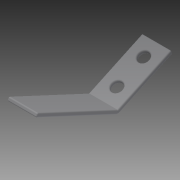
# Autodesk Inventor part: small rail
Saved by Autodesk Inventor 2014 SP1 (Build 180222100, 222)
## iProperties
Created: 2013-11-15
Part Number: small rail
Material: Polycarbonate, Clear
Document SubType Name: Modeling
Designer: RyanHughes
Density: 1.2 g/cm^3
Appearance: Polycarbonate - Clear
Author: RyanHughes
Autodesk Inventor part; units mm, degrees
ref_plane "YZ Plane" through (0, 0, 0) normal (1, 0, 0) x (0, 1, 0)
ref_plane "XZ Plane" through (0, 0, 0) normal (0, 1, 0) x (-1, 0, 0)
ref_plane "XY Plane" through (0, 0, 0) normal (0, 0, 1) x (1, 0, 0)
sketch "Sketch1" plane through (0, 0, 0) normal (0, 1, 0) x (-1, 0, 0)
  line L0 (6.35, -31.75) -> (-6.35, -31.75)
  line L1 (-6.35, -31.75) -> (-6.35, 31.75)
  line L2 (-6.35, 31.75) -> (6.35, 31.75)
  line L3 (6.35, 31.75) -> (6.35, -31.75)
  line L4 (6.35, -31.75) -> (-6.35, 31.75) construction
  line L5 (-6.35, -31.75) -> (6.35, 31.75) construction
  point P0 (0, 0)
  dimension "d0" = 12.7
  dimension "d1" = 63.5
  constraints: 12 end point, 2 midpoint, 2 parallel, 1 horizontal, 1 perpendicular
  measures "d0" distance of L1.end L2.end
  measures "d1" distance of L0.end L1.end
extrude "Extrusion1" add sketch "Sketch1" along normal blind 1.5875
sketch "Sketch2" plane through (0, 1.5875, 0) normal (0, 1, 0) x (1, 0, 0)
  line L0 (6.35, 31.75) -> (-6.35, 31.75) projected
  line L1 (6.35, -31.75) -> (6.35, 31.75) projected
  circle A0 centre (0, 25.4) radius 2.2225
  circle A1 centre (0, 12.7) radius 2.2225
  point P0 (0, 0)
  dimension "d4" = 4.445
  dimension "d5" = 6.35
  dimension "d8" = 12.7
  constraints: 2 centre point, 1 vertical, 2 other
  measures "d4" diameter of A0
  measures "d5" distance from line of A0.centre L0
  measures "d8" distance of A0.centre A1.centre
extrude "Extrusion2" cut sketch "Sketch2" against normal blind 1.5875
sketch "Sketch3" plane through (0, 1.5875, 0) normal (0, 1, 0) x (1, 0, 0)
  circle A0 centre (0, 12.7) radius 2.2225 projected
  line L0 (-6.35, 31.75) -> (-6.35, -31.75) projected
  line L1 (6.35, -31.75) -> (6.35, 31.75) projected
  line L2 (6.35, 6.35) -> (-6.35, 6.35)
  point P0 (0, 0)
  dimension "d15" = 6.35
  constraints: 2 end point, 2 point on line, 1 perpendicular
  measures "d15" distance from line of L2 A0.centre
bend part "Bend Part1" radius 0.2911 angle 50 line through (6.35, 1.5875, -6.35) along (-1, 0, 0) centre toward (0, 1, 0) moving side (0, 0, 1) both sides yes
fillet "Fillet1" radius 0.508 23 edges at (6.35, 6.9552, -17.9256) (0, 12.2956, -29.3781) (-6.35, 6.9552, -17.9256) (6.35, 1.5875, -6.35) (6.35, 9.6388, 10.9806) (-6.35, 1.5875, -6.35) (-6.35, 9.6388, 10.9806) (-6.35, 5.5164, -18.5965) (0, 10.8568, -30.049) (6.35, 5.5164, -18.5965) (-6.35, 0, -6.35) (-6.35, 8.2, 11.6515) (6.35, 0, -6.35) (6.35, 8.2, 11.6515) (6.35, 11.5762, -29.7136) (6.35, 16.9435, 28.5237) (-6.35, 16.9435, 28.5237) (0, 17.6629, 28.1882) (0, 16.2241, 28.8591) (-2.2225, 9.612, -23.6231) (-2.2225, 8.1732, -24.294) (-2.2225, 4.2447, -12.113) (-2.2225, 2.806, -12.7839)
body "Solid1"
